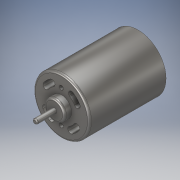
# Autodesk Inventor part: Moteur
Saved by Autodesk Inventor 2019 (Build 230136000, 136)
## iProperties
Created: 2019-07-29
Part Number: Moteur
Material: Acier inoxydable
Document SubType Name: Modeling
Designer: Sébastien DI MERCURIO
Mass: 178.187 g
Surface Area: 44.2768 cm^2
Volume: 22.2734 cm^3
Density: 8 g/cm^3
Appearance: Semi-poli
Author: Sébastien DI MERCURIO
Autodesk Inventor part; units mm, degrees
ref_plane "YZ Plane" through (0, 0, 0) normal (1, 0, 0) x (0, 1, 0)
ref_plane "XZ Plane" through (0, 0, 0) normal (0, 1, 0) x (-1, 0, 0)
ref_plane "XY Plane" through (0, 0, 0) normal (0, 0, 1) x (1, 0, 0)
sketch "Esquisse1" plane through (0, 0, 0) normal (0, 0, 1) x (1, 0, 0)
  circle A0 centre (0, 0) radius 13.75
  dimension "d0" = 27.5
  constraints: 1 centre point, 1 coincident
  measures "d0" diameter of A0
extrude "Extrusion1" add sketch "Esquisse1" along normal blind 37.5
sketch "Esquisse2" plane through (0, 0, 0) normal (0, 0, -1) x (-1, 0, 0)
  circle A0 centre (0, 0) radius 5
  dimension "d3" = 10
  constraints: 1 centre point, 1 coincident
  measures "d3" diameter of A0
extrude "Extrusion2" add sketch "Esquisse2" along normal blind 3.5
sketch "Esquisse3" plane through (0, 0, 37.5) normal (0, 0, 1) x (1, 0, 0)
  circle A0 centre (0, 0) radius 1.2
  dimension "d6" = 2.4
  constraints: 1 centre point, 1 coincident
  measures "d6" diameter of A0
extrude "Extrusion3" add sketch "Esquisse3" along normal blind 13
sketch "Esquisse4" plane through (0, 0, 37.5) normal (0, 0, 1) x (1, 0, 0)
  circle A0 centre (0, 0) radius 1.2 projected
  circle A1 centre (0, 0) radius 5
  dimension "d9" = 10
  constraints: 1 centre point, 1 coincident
  measures "d9" diameter of A1
extrude "Extrusion4" add sketch "Esquisse4" along normal blind 3.5
fillet "Congé1" radius 1 2 edges at (-5, 0, 41) (5, 0, -3.5)
fillet "Congé2" radius 1 1 edges at (-13.75, 0, 37.5)
fillet "Congé3" radius 0.5 1 edges at (-1.2, 0, 50.5)
sketch "Esquisse5" plane through (0, 0, 37.5) normal (0, 0, 1) x (1, 0, 0)
  circle A0 centre (0, 8) radius 1
  arc A1 (7.7336, 4.6035) -> (4.9749, 7.5) centre (0, 0) ccw construction
  arc A2 (9.0225, 5.3707) -> (5.8041, 8.75) centre (0, 0) ccw
  arc A3 (6.4446, 3.8362) -> (4.1458, 6.25) centre (0, 0) ccw
  arc A4 (6.4446, 3.8362) -> (9.0225, 5.3707) centre (7.7336, 4.6035) ccw
  arc A5 (5.8041, 8.75) -> (4.1458, 6.25) centre (4.9749, 7.5) ccw
  line L0 (0, 0) -> (0, 21.7918) construction
  circle A6 centre (0, -8) radius 1
  arc A7 (8.75, -5.8041) -> (6.25, -4.1458) centre (7.5, -4.9749) ccw
  arc A8 (5.3707, -9.0225) -> (8.75, -5.8041) centre (0, 0) ccw
  arc A9 (3.8362, -6.4446) -> (5.3707, -9.0225) centre (4.6035, -7.7336) ccw
  arc A10 (3.8362, -6.4446) -> (6.25, -4.1458) centre (0, 0) ccw
  arc A11 (-5.8041, -8.75) -> (-4.1458, -6.25) centre (-4.9749, -7.5) ccw
  arc A12 (-9.0225, -5.3707) -> (-5.8041, -8.75) centre (0, 0) ccw
  arc A13 (-6.4446, -3.8362) -> (-9.0225, -5.3707) centre (-7.7336, -4.6035) ccw
  arc A14 (-6.4446, -3.8362) -> (-4.1458, -6.25) centre (0, 0) ccw
  arc A15 (-8.75, 5.8041) -> (-6.25, 4.1458) centre (-7.5, 4.9749) ccw
  arc A16 (-5.3707, 9.0225) -> (-8.75, 5.8041) centre (0, 0) ccw
  arc A17 (-3.8362, 6.4446) -> (-5.3707, 9.0225) centre (-4.6035, 7.7336) ccw
  arc A18 (-3.8362, 6.4446) -> (-6.25, 4.1458) centre (0, 0) ccw
  dimension "d15" = 2
  dimension "d16" = 3
  dimension "d17" = 8
  dimension "d19" = 7
  dimension "d21" = 5
  dimension "d22" = 9
  dimension "d25" = 360
  dimension "d29" = 360
  constraints: 34 point on circle, 19 centre point, 4 tangent, 3 coincident, 2 end point, 1 point on line, 1 vertical, 50 other
  measures "d15" diameter of A0
  measures "d16" radial gap between concentric circles of A3 A2
  measures "d17" distance of point (0, 0) A0.centre
  measures "d21" distance of A1.end A0.centre
  measures "d22" distance of A1.start L0.start
extrude "Extrusion5" cut sketch "Esquisse5" against normal blind 5
